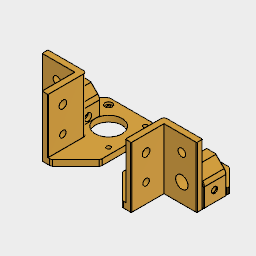
XY_Stepper_Mount_1.0_F01 (Autodesk Fusion 360 design; units mm, degrees)
Autodesk Fusion 360 part; units mm, degrees
sketch "スケッチ1" plane through (0, 0, 0) normal (0, 0, 1) x (1, 0, 0)
  circle A0 centre (0, 0) radius 11.2
  line L0 (-35, 21) -> (21, 21)
  line L1 (21, 21) -> (21, -48.5)
  line L2 (21, -48.5) -> (-35, -48.5)
  line L3 (-35, -48.5) -> (-35, 21)
  line L4 (-35, 21) -> (21, -48.5) construction
  line L5 (21, 21) -> (-35, -48.5) construction
  line L6 (-35, -21) -> (-7.5, -21)
  line L7 (-7.5, -21) -> (-7.5, -48.5)
  line L8 (0, -48.5) -> (21, -27.5)
  line L9 (-35, 5) -> (-25.5, 5)
  line L10 (-25.5, 5) -> (-25.5, 4)
  line L11 (-25.5, 4) -> (-35, 4)
  line L12 (-35, -15) -> (-25.5, -15)
  line L13 (-25.5, -15) -> (-25.5, -16)
  line L14 (-25.5, -16) -> (-35, -16)
  line L15 (-25.5, 4) -> (-25.5, -15)
  line L16 (-26.5, 4) -> (-26.5, -15)
  line L17 (-25.5, 4) -> (-11.2, 4)
  line L18 (-11.2, 4) -> (-11.2, -16)
  line L19 (-11.2, -16) -> (-25.5, -16)
  line L20 (-11.2, -16) -> (-2.5, -16)
  line L21 (-2.5, -16) -> (-2.5, -48.5)
  circle A1 centre (15.5, 15.5) radius 1.75
  circle A2 centre (15.5, -15.5) radius 1.75
  circle A3 centre (-15.5, 15.5) radius 1.75
  circle A4 centre (-15.5, 15.5) radius 3.05
  point P0 (-7, -13.75)
  dimension "d1" = 22.4
  dimension "d2" = 69.5
  dimension "d3" = 56
  dimension "d4" = 21
  dimension "d5" = 21
  dimension "d6" = 27.5
  dimension "d7" = 27.5
  dimension "d8" = 21
  dimension "d9" = 21
  dimension "d10" = 5
  dimension "d11" = 1
  dimension "d12" = 19
  dimension "d13" = 1
  dimension "d14" = 9.5
  dimension "d15" = 1
  dimension "d16" = 5
  dimension "d17" = 3.5
  dimension "d18" = 3.5
  dimension "d19" = 3.5
  dimension "d20" = 15.5
  dimension "d21" = 15.5
  dimension "d22" = 15.5
  dimension "d23" = 15.5
  dimension "d24" = 15.5
  dimension "d25" = 15.5
  dimension "d26" = 6.1
  measures "d1" diameter of A0
  measures "d2" distance of L0.end L1.end
  measures "d3" distance of L1.end L2.end
  measures "d4" distance of A0.centre L1
  measures "d5" distance of A0.centre L0
  measures "d6" distance of L6.start L6.end
  measures "d7" distance of L6.end L7.end
  measures "d8" distance of L2 L8.end
  measures "d9" distance of L1.end L8.start
  measures "d10" distance of L6 L14
  measures "d11" distance of L12 L14
  measures "d12" distance of L11 L12
  measures "d13" distance of L9 L11
  measures "d14" distance of L9.start L9.end
  measures "d15" distance of L15 L16
  measures "d16" distance of L7 L21
  measures "d17" diameter of A1
  measures "d18" diameter of A2
  measures "d19" diameter of A3
  measures "d20" distance of A0.centre A1.centre
  measures "d21" distance of A0.centre A2.centre
  measures "d22" distance of A0.centre A2.centre
  measures "d23" distance of A0.centre A1.centre
  measures "d24" distance of A0.centre A3.centre
  measures "d25" distance of A0.centre A3.centre
  measures "d26" diameter of A4
extrude "押し出し1" add sketch "スケッチ1" along normal blind 5 contours L0 L1 L2 L3 L8 L9 L10 L17 L18 L20 L21 | L13 L15 L17 L18 L19 | L2 L3 L6 L7 L14 L19 L20 L21 | L3 L9 L10 L11 | L11 L12 L15 L16 | L3 L12 L13 L14 | L3 L11 L12 L16 makes body 1
extrude "押し出し2" add sketch "スケッチ1" along normal blind 3 contours A4 bodies 1
extrude "押し出し3" add sketch "スケッチ1" along normal blind 51 contours L2 L3 L6 L7 L14 L19 L20 L21 bodies 1
extrude "押し出し4" add sketch "スケッチ1" along normal blind 26 contours L13 L15 L17 L18 L19 | L11 L12 L15 L16 | L3 L12 L13 L14 | L3 L11 L12 L16 bodies 1
chamfer "面取り1" distance 14.5 angle 45 1 edges at (-35, 21, 2.5) on bodies 1
chamfer "面取り2" distance 5 angle 45 1 edges at (21, 21, 2.5) on bodies 1
sketch "スケッチ2" plane through (0, 4, 0) normal (0, 1, 0) x (-1, 0, 0)
  line L0 (11.2, 5) -> (35, 5)
  line L1 (35, 5) -> (35, 26)
  line L2 (35, 26) -> (11.2, 26)
  line L3 (11.2, 26) -> (11.2, 5)
  circle A0 centre (22.5, 16) radius 5.2
  dimension "d37" = 10.4
  dimension "d38" = 10
  dimension "d39" = 12.5
  measures "d37" diameter of A0
  measures "d38" distance of L2 A0.centre
  measures "d39" distance of L1 A0.centre
extrude "押し出し5" cut sketch "スケッチ2" against normal blind 30 contours A0 bodies 1
chamfer "面取り3" distance 7.2 angle 45 1 edges at (-11.2, -6, 26) on bodies 1
chamfer "面取り4" distance 8.4 angle 45 1 edges at (-35, -6, 26) on bodies 1
extrude "押し出し6" cut sketch "スケッチ1" along normal blind 19.6 contours L3 L12 L13 L14 bodies 1
extrude "押し出し7" cut sketch "スケッチ1" along normal blind 15 contours L3 L9 L10 L11 | L11 L12 L15 L16 bodies 1
chamfer "面取り5" distance 4.8973 angle 54 1 edges at (-33, -15.5, 19.6) measured on face at (-31.5333, -2.3333, 21.0667) on bodies 1
sketch "スケッチ3" plane through (0, -21, 0) normal (0, -1, 0) x (1, 0, 0)
  circle A0 centre (-22.5, 16) radius 5.2
  line L0 (-35, 0) -> (-7.5, 0)
  line L1 (-7.5, 0) -> (-7.5, 51)
  line L2 (-7.5, 51) -> (-35, 51)
  line L3 (-35, 51) -> (-35, 0)
  circle A1 centre (-22.5, 37.5) radius 3.2
  circle A2 centre (-22.5, 37.5) radius 4.75 construction
  dimension "d50" = 6.4
  dimension "d51" = 13.5
  dimension "d52" = 12.5
  dimension "d87" = 9.5
  measures "d50" diameter of A1
  measures "d51" distance of L2 A1.centre
  measures "d52" distance of L3 A1.centre
  measures "d87" diameter of A2
extrude "押し出し8" cut sketch "スケッチ3" against normal blind 10 contours A1 bodies 1
sketch "スケッチ4" plane through (-7.5, 0, 0) normal (-1, 0, 0) x (0, -1, 0)
  line L0 (21, 0) -> (48.5, 0)
  line L1 (48.5, 0) -> (48.5, 51)
  line L2 (48.5, 51) -> (21, 51)
  line L3 (21, 51) -> (21, 0)
  circle A0 centre (36, 37.5) radius 3.2
  circle A1 centre (36, 16) radius 2.7
  dimension "d55" = 6.4
  dimension "d56" = 5.4
  dimension "d57" = 12.5
  dimension "d58" = 12.5
  dimension "d59" = 13.5
  dimension "d60" = 16
  measures "d55" diameter of A0
  measures "d56" diameter of A1
  measures "d57" distance of L1 A0.centre
  measures "d58" distance of L1 A1.centre
  measures "d59" distance of L2 A0.centre
  measures "d60" distance of L0 A1.centre
extrude "押し出し9" cut sketch "スケッチ4" against normal blind 10 contours A0 | A1 bodies 1
sketch "スケッチ5" plane through (-35, 0, 0) normal (-1, 0, 0) x (0, -1, 0)
  line L0 (-4, 17.6) -> (-4, 0)
  line L1 (-4, 0) -> (15, 0)
  line L2 (15, 0) -> (15, 17.6)
  line L3 (15, 17.6) -> (-4, 17.6)
  circle A0 centre (6, 9) radius 1.75
  circle A1 centre (6, 9) radius 2.5
  circle A2 centre (6, 9) radius 2.35
  dimension "d63" = 3.5
  dimension "d64" = 10
  dimension "d65" = 9
  dimension "d66" = 5
  dimension "d67" = 4.7
  measures "d63" diameter of A0
  measures "d64" distance of L0 A0.centre
  measures "d65" distance of L1 A0.centre
  measures "d66" diameter of A1
  measures "d67" diameter of A2
extrude "押し出し10" cut sketch "スケッチ5" against normal blind 30 contours A0 bodies 1
extrude "押し出し11" cut sketch "スケッチ5" against normal blind 5 contours A2 bodies 1
extrude "押し出し12" cut sketch "スケッチ5" against normal blind 1 contours A1 bodies 1
sketch "スケッチ6" plane through (-11.2, 0, 0) normal (1, 0, 0) x (0, 1, 0)
  circle A0 centre (-6, 9) radius 1.75
  line L0 (4, 18.8) -> (-16, 18.8)
  line L1 (-16, 18.8) -> (-16, 5)
  line L2 (-16, 5) -> (0, 5)
  line L3 (0, 5) -> (4, 5)
  line L4 (4, 5) -> (4, 18.8)
  circle A1 centre (-6, 9) radius 3
  dimension "d74" = 6
  measures "d74" diameter of A1
extrude "押し出し13" cut sketch "スケッチ6" against normal blind 3 contours A1 bodies 1
fillet "フィレット1" radius 2.5 1 edges at (-2.5, -16, 28) on bodies 1
fillet "フィレット2" radius 2.5 6 edges at (0, -48.5, 2.5) (21, -27.5, 2.5) (21, 16, 2.5) (16, 21, 2.5) (-20.5, 21, 2.5) (-35, 6.5, 2.5) on bodies 1
fillet "フィレット3" radius 5 2 edges at (-11.2, -6, 18.8) (-35, -5.5, 17.6) on bodies 1
fillet "フィレット4" radius 0.5 4 edges at (-35, -16, 25.5) (-35, -21, 25.5) (-7.5, -48.5, 25.5) (-2.5, -48.5, 28) on bodies 1
fillet "フィレット5" radius 0.5 9 edges at (-11.2, 4, 10.8645) (-11.5806, 4, 18.6423) (-15.5322, 4, 23.1322) (-30.0678, 4, 22.5322) (-34.6194, 4, 17.4423) (-35, 4, 7.7645) (-35, -15, 7.7645) (-34.6194, -15, 17.4423) (-31.5363, -15, 21.0637) on bodies 1
fillet "フィレット6" radius 0.5 4 edges at (-26.5, 4, 6.3387) (-25.5, 4, 8.3763) (-25.5, -6, 11.7526) (-26.5, -5.5, 12.6774) on bodies 1
fillet "フィレット7" radius 0.5 1 edges at (-35, 5, 2.5) on bodies 1
fillet "フィレット8" radius 0.5 1 edges at (-26.5, -15, 6.2507) on bodies 1
ref_plane "作業平面1" through (30, 0, 0) normal (1, 0, 0) x (0, 1, 0)
mirror "ミラー1" about plane through (30, 0, 0) normal (1, 0, 0) of bodies 1 makes body 2
